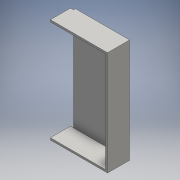
# Autodesk Inventor part: LEDs_protect
Saved by Autodesk Inventor 2016 (Build 200138000, 138)
## iProperties
Created: 2015-10-21
Part Number: LEDs_protect
Material: Generic
Document SubType Name: Modeling
Designer: fei
Density: 1 g/cm^3
Appearance: Default
Author: fei
Autodesk Inventor part; units mm, degrees
ref_plane "YZ Plane" through (0, 0, 0) normal (1, 0, 0) x (0, 1, 0)
ref_plane "XZ Plane" through (0, 0, 0) normal (0, 1, 0) x (-1, 0, 0)
ref_plane "XY Plane" through (0, 0, 0) normal (0, 0, 1) x (1, 0, 0)
sketch "Sketch1" plane through (0, 0, 0) normal (1, 0, 0) x (0, 1, 0)
  line L0 (10, 52) -> (-10, 52)
  line L1 (-10, 52) -> (-10, -52)
  line L2 (-10, -52) -> (10, -52)
  line L3 (10, -52) -> (10, 52)
  point P0 (0, 0)
  dimension "d0" = 104
  dimension "d1" = 20
  dimension "d2" = 52
  dimension "d3" = 10
  constraints: 8 end point, 2 parallel, 1 horizontal, 1 perpendicular
  measures "d0" distance of L2.end L0.start
  measures "d1" distance of L1.end L2.end
  measures "d2" distance from line of L2 point (0, 0)
  measures "d3" distance from line of L3 point (0, 0)
extrude "Extrusion1" add sketch "Sketch1" against normal blind 2
sketch "Sketch2" plane through (-2, 0, 0) normal (-1, 0, 0) x (0, 0, 1)
  line L0 (52, 10) -> (-52, 10) projected
  line L1 (-52, -10) -> (52, -10) projected
  line L2 (-52, 10) -> (-50, 10)
  line L3 (-50, 10) -> (-50, -10)
  line L4 (-50, -10) -> (-52, -10)
  line L5 (-52, -10) -> (-52, 10)
  line L6 (52, -10) -> (52, 10) projected
  line L7 (52, 10) -> (50, 10)
  line L8 (50, 10) -> (50, -10)
  line L9 (50, -10) -> (52, -10)
  line L10 (52, -10) -> (52, 10)
  point P0 (0, 0)
  dimension "d6" = 2
  dimension "d7" = 2
  constraints: 16 end point, 4 parallel, 2 horizontal, 2 perpendicular, 2 point on line
  measures "d6" distance between parallel lines of L5 L3
  measures "d7" distance between parallel lines of L6 L8
extrude "Extrusion2" add sketch "Sketch2" along normal blind 55 contours L6 L1 L8 L0 | L3 L1 L5 L0
sketch "Sketch3" plane through (0, 0, 0) normal (1, 0, 0) x (0, 0, -1)
  line L0 (52, 10) -> (-52, 10) projected
  line L1 (52, 10) -> (-52, 10)
  line L2 (-52, 10) -> (-52, 12)
  line L3 (-52, 12) -> (52, 12)
  line L4 (52, 12) -> (52, 10)
  line L5 (-52, 10) -> (-52, -10) projected
  point P0 (0, 0)
  dimension "d10" = 2
  dimension "d11" = 0
  constraints: 8 end point, 2 parallel, 1 horizontal, 1 perpendicular
  measures "d10" distance between parallel lines of L3 L0
  measures "d11" distance between parallel lines of L5 L2
extrude "Extrusion3" add sketch "Sketch3" against normal blind 54
body "Solid1"
